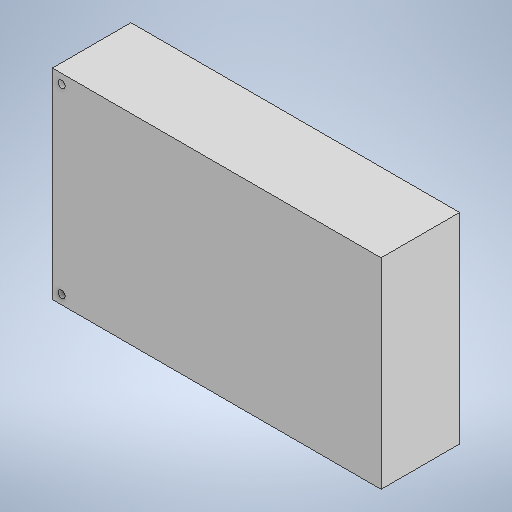
# Autodesk Inventor part: SMPS
Saved by Autodesk Inventor 2025 (Build 290162000, 162)
## iProperties
Created: 2024-06-01
Part Number: SMPS
Material: 일반
Document SubType Name: Modeling
Designer: ckhye
Density: 1 g/cm^3
Appearance: 기본값
Author: ckhye
Autodesk Inventor part; units mm, degrees
ref_plane "YZ Plane" through (0, 0, 0) normal (1, 0, 0) x (0, 1, 0)
ref_plane "XZ Plane" through (0, 0, 0) normal (0, 1, 0) x (-1, 0, 0)
ref_plane "XY Plane" through (0, 0, 0) normal (0, 0, 1) x (1, 0, 0)
sketch "스케치1" plane through (0, 0, 0) normal (0, 0, 1) x (1, 0, 0)
  line L0 (-79.5, 48.5) -> (79.5, 48.5)
  line L1 (79.5, 48.5) -> (79.5, -48.5)
  line L2 (79.5, -48.5) -> (-79.5, -48.5)
  line L3 (-79.5, -48.5) -> (-79.5, 48.5)
  line L4 (-79.5, 48.5) -> (79.5, -48.5) construction
  line L5 (79.5, 48.5) -> (-79.5, -48.5) construction
  line L6 (-91.9522, 44) -> (117.9922, 44) construction
  line L7 (-91.9522, -44) -> (123.3329, -44) construction
  line L8 (-75, 56.2036) -> (-75, -62.2124) construction
  circle A0 centre (-75, 44) radius 1.75
  circle A1 centre (-75, -44) radius 1.75
  point P0 (0, 0)
  dimension "d0" = 159
  dimension "d1" = 97
  dimension "d2" = 4.5
  dimension "d3" = 4.5
  dimension "d4" = 4.5
  dimension "d5" = 3.5
  dimension "d6" = 3.5
  constraints: 18 end point, 4 point on line, 3 horizontal, 2 centre point, 2 midpoint, 2 parallel, 1 perpendicular, 1 vertical
  measures "d0" distance of L1.end L2.end
  measures "d1" distance between parallel lines of L2 L0
  measures "d2" distance between parallel lines of L6 L0
  measures "d3" distance between parallel lines of L3 L8
  measures "d4" distance between parallel lines of L2 L7
  measures "d5" diameter of A0
  measures "d6" diameter of A1
extrude "돌출1" add sketch "스케치1" along normal blind 38
